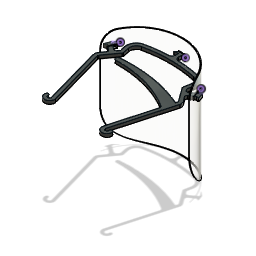
Full_Face_Shield_2.1 (Autodesk Fusion 360 design; units mm, degrees)
Autodesk Fusion 360 part; units mm, degrees
note: some values were not read from the file. Chosen so that the rebuilt part matches the saved one: which face or edge a step refers to; which pieces of a blend or face edit are solid. Set by a fixed rule: which sketch regions a step uses.
(part 1 of 2)
sketch "Sketch1" plane through (0, 0, 0) normal (0, 1, 0) x (1, 0, 0)
  line L0 (0, 0) -> (150, 0) construction
  line L1 (150, 0) -> (150, 165) construction
  line L2 (0, 165) -> (0, 0) construction
  line L3 (75, 0) -> (110, 0) construction
  line L4 (75, 0) -> (40, 0) construction
  line L5 (150, 165) -> (150, 115)
  line L6 (0, 165) -> (0, 115) construction
  line L7 (75, 165) -> (15, 165) construction
  line L8 (16.018879, 159.905605) -> (19.543063, 142.284685)
  line L9 (18.544504, 138.180629) -> (1.725632, 117.15704)
  line L10 (77.5, 165) -> (135, 165)
  line L11 (133.981121, 159.905605) -> (130.456937, 142.284685)
  line L12 (131.455496, 138.180629) -> (148.274368, 117.15704)
  arc A0 (20.165444, 165.82865) -> (16.018879, 159.905605) centre (20.921782, 160.886186) ccw
  arc A1 (133.981121, 159.905605) -> (129.834556, 165.82865) centre (129.078218, 160.886186) ccw
  arc A2 (18.544504, 138.180629) -> (19.543063, 142.284685) centre (14.64016, 141.304105) ccw
  arc A3 (130.456937, 142.284685) -> (131.455496, 138.180629) centre (135.35984, 141.304105) ccw
  arc A4 (1.725632, 117.15704) -> (0.907492, 112.390961) centre (5.629976, 114.033564) ccw
  arc A5 (149.092508, 112.390961) -> (148.274368, 117.15704) centre (144.370024, 114.033564) ccw
  arc A6 (-2.178712, 120.280515) -> (-3.814992, 110.748358) centre (5.629976, 114.033564) ccw
  line L13 (14.64016, 141.304105) -> (-2.178712, 120.280515)
  line L14 (11.115976, 158.925025) -> (14.64016, 141.304105)
  arc A7 (19.409105, 170.771114) -> (11.115976, 158.925025) centre (20.921782, 160.886186) ccw
  arc A8 (130.590895, 170.771114) -> (19.409105, 170.771114) centre (75, -192.5) ccw
  arc A9 (138.884024, 158.925025) -> (130.590895, 170.771114) centre (129.078218, 160.886186) ccw
  line L15 (138.884024, 158.925025) -> (135.35984, 141.304105)
  line L16 (135.35984, 141.304105) -> (152.178712, 120.280515)
  arc A10 (153.814992, 110.748358) -> (152.178712, 120.280515) centre (144.370024, 114.033564) ccw
  line L17 (75, 170) -> (75, 165) construction
  arc A11 (29.826985, 93.888373) -> (50.996347, 169.204402) centre (0.850567, 142.665976) ccw
  arc A12 (42.173763, 96.800594) -> (56.437117, 169.524404) centre (0.850567, 142.665976) ccw
  arc A13 (99.003653, 169.204402) -> (120.173015, 93.888373) centre (149.149433, 142.665976) ccw
  arc A14 (93.562883, 169.524404) -> (107.826237, 96.800594) centre (149.149433, 142.665976) ccw
  circle A15 centre (1.813222, 102.177115) radius 2.5
  circle A16 centre (148.186778, 102.177115) radius 2.5
  line L18 (-3.814992, 110.748358) -> (0, 99.780255)
  line L19 (0.907492, 112.390961) -> (4.174464, 102.998416)
  line L20 (149.092508, 112.390961) -> (145.825536, 102.998416)
  line L21 (153.814992, 110.748358) -> (150, 99.780255)
  arc A17 (145.355882, 79.248283) -> (4.644118, 79.248283) centre (75, -70) ccw
  line L22 (-2.880043, 72.125873) -> (30, -50)
  arc A18 (30, -50) -> (34.828079, -48.700133) centre (32.414039, -49.350066) ccw
  arc A19 (2.512122, 83.770958) -> (-2.880043, 72.125873) centre (6.776115, 74.725608) ccw
  arc A20 (4.644118, 79.248283) -> (1.948036, 73.42574) centre (6.776115, 74.725608) ccw
  line L23 (1.948036, 73.42574) -> (34.828079, -48.700133)
  arc A21 (29.826985, 93.888373) -> (2.512122, 83.770958) centre (75, -70) ccw
  arc A22 (147.487878, 83.770958) -> (120.173015, 93.888373) centre (75, -70) ccw
  arc A23 (50.996347, 169.204402) -> (20.165444, 165.82865) centre (75, -192.5) ccw
  arc A24 (129.834556, 165.82865) -> (99.003653, 169.204402) centre (75, -192.5) ccw
  line L24 (77.5, 170) -> (77.5, 165)
  line L25 (72.5, 165) -> (72.5, 100)
  line L26 (72.5, 100) -> (72.5, 99.500001)
  line L27 (72.5, 99.500001) -> (72.000001, 99.500001)
  line L28 (72.000001, 99.500001) -> (71.807399, 99.500001)
  line L29 (77.5, 165) -> (77.5, 99.500001)
  line L30 (72.5, 165) -> (72.5, 170.500003)
  line L31 (77.5, 169.991379) -> (77.5, 170.500003)
  arc A25 (93.562883, 169.524404) -> (77.5, 169.991379) centre (75, -192.5) ccw
  arc A26 (72.5, 169.991379) -> (56.437117, 169.524404) centre (75, -192.5) ccw
  line L32 (150, 165) -> (77.5, 165) construction
  line L33 (75, 165) -> (0, 165) construction
  arc A27 (107.826237, 96.800594) -> (77.5, 99.981617) centre (75, -70) ccw
  arc A28 (72.5, 99.981617) -> (42.173763, 96.800594) centre (75, -70) ccw
  arc A29 (152.880043, 72.125873) -> (147.487878, 83.770958) centre (143.223885, 74.725608) ccw
  arc A30 (148.051964, 73.42574) -> (145.355882, 79.248283) centre (143.223885, 74.725608) ccw
  line L34 (148.051964, 73.42574) -> (115.171921, -48.700133)
  line L35 (152.880043, 72.125873) -> (120, -50)
  arc A31 (145.355882, 79.248283) -> (4.644118, 79.248283) centre (75, -70) ccw
  arc A32 (115.171921, -48.700133) -> (120, -50) centre (117.585961, -49.350066) ccw
  dimension "d1" = 150
  dimension "d2" = 165
  dimension "d3" = 35
  dimension "d4" = 35
  dimension "d5" = 50
  dimension "d6" = 50
  dimension "d7" = 60
  dimension "d8" = 60
  dimension "d9" = 5
  dimension "d14" = 10
  dimension "d15" = -2.5
  constraint horizontal L0
  constraint vertical L1
  constraint horizontal L32
  constraint vertical L2
  constraint coincident L0.start L2.end
  constraint midpoint L0 L3.start
  constraint parallel L0 L3
  constraint parallel L0 L4
  constraint perpendicular L5 L32
  constraint perpendicular L6 L32
  constraint parallel L7 L32
  constraint parallel L10 L32
  constraint coincident L7.end L8
  constraint coincident L7.end A24
  constraint tangent A0 A24
  constraint tangent L8 A0
  constraint coincident L10.end L11
  constraint coincident L10.end A24
  constraint tangent A1 A24
  constraint tangent L11 A1
  constraint equal A0 A1
  constraint tangent L8 A2
  constraint tangent L9 A2
  constraint equal A0 A2
  constraint tangent L11 A3
  constraint tangent L12 A3
  constraint equal A0 A3
  constraint coincident L6.end L9
  constraint coincident L6.end L19
  constraint tangent L9 A4
  constraint tangent A4 L19
  constraint equal A0 A4
  constraint coincident L5.end L12
  constraint coincident L5.end L20
  constraint tangent L12 A5
  constraint tangent A5 L20
  constraint equal A0 A5
  constraint perpendicular L17 L32
  constraint symmetric L17 A11 A13
  constraint symmetric L17 A12 A14
  constraint tangent A15 L19
  constraint symmetric L17 A15 A16
  constraint parallel L18 L19
  constraint concentric A4 A6
  constraint parallel L9 L13
  constraint parallel L8 L14
  constraint concentric A0 A7
  constraint concentric A8 A24
  constraint concentric A1 A9
  constraint parallel L11 L15
  constraint parallel L12 L16
  constraint concentric A5 A10
  constraint parallel L20 L21
  constraint tangent A6 L18
  constraint tangent L14 A7
  constraint tangent A7 A8
  constraint tangent A6 L13
  constraint tangent A9 L15
  constraint tangent A8 A9
  constraint tangent L16 A10
  constraint tangent A10 L21
  constraint concentric A17 A22
  constraint tangent A19 A22
  constraint tangent L22 A19
  constraint concentric A11 A12
  constraint concentric A21 A22
  constraint concentric A19 A20
  constraint parallel L22 L23
  constraint tangent A20 L23
  constraint concentric A22 A27
  constraint concentric A23 A24
  constraint coincident L17.start A24
  constraint concentric A24 A25
  constraint parallel L25 L26
  constraint perpendicular L26 L27
  constraint perpendicular L26 L28
  constraint perpendicular L27 L29
  constraint parallel L25 L30
  constraint parallel L25 L31
  constraint concentric A25 A26
  constraint collinear L32 L33
  constraint coincident L7.start L32
  constraint concentric A27 A28
  constraint symmetric L17 L22.end L35.end
  constraint symmetric L17 A19 A29
  constraint symmetric L17 A20 A30
  constraint tangent L35 A32
  measures "d1" distance of L0.start L0.end
  measures "d2" distance of L0.start L2.start
  measures "d3" distance of L3.start L3.end
  measures "d4" distance of L3.start L4.end
  measures "d5" distance of L1.end L5.end
  measures "d6" distance of L2.start L6.end
  measures "d7" distance of L7.start L7.end
  measures "d8" distance of L7.start L10.end
  measures "d9" radius of A0
  measures "d14" radius of A19
sketch "Sketch2" plane through (0, 0, 0) normal (0, 1, 0) x (1, 0, 0)
  arc A0 (74.500001, 175.000338) -> (20, 171.000003) centre (74.500001, -198.250003) ccw
  arc A1 (74.500001, 170.000338) -> (20.730073, 166.05359) centre (74.500001, -198.250003) ccw
  arc A2 (20, 171.000003) -> (11, 159.000002) centre (20.833334, 161.000002) ccw
  line L0 (11, 159.000002) -> (14.161452, 143.4562)
  line L1 (13.13349, 139.295831) -> (-1, 122.000002)
  arc A3 (-1, 122.000002) -> (-3.968884, 110.553272) centre (7.879032, 113.588711) ccw
  line L2 (0.330661, 92.053201) -> (30, -50)
  arc A4 (0.330661, 92.053201) -> (-3.968884, 110.553272) centre (-413.734399, 5.571259) ccw
  arc A5 (30, -50) -> (34.894386, -48.977755) centre (32.447193, -49.488877) ccw
  arc A6 (114.105616, -48.977755) -> (119.000002, -50) centre (116.552809, -49.488877) ccw
  arc A7 (13.13349, 139.295831) -> (14.161452, 143.4562) centre (9.261768, 142.459654) ccw
  arc A8 (20.415228, 166.017274) -> (15.899683, 159.996548) centre (20.833334, 161.000002) ccw
  line L3 (15.899683, 159.996548) -> (19.061135, 144.452745)
  arc A9 (17.005211, 136.132009) -> (19.061135, 144.452745) centre (9.261768, 142.459654) ccw
  line L4 (17.005211, 136.132009) -> (2.74065, 118.675781)
  arc A10 (2.74065, 118.675781) -> (0.87468, 111.794195) centre (7.879032, 113.588711) ccw
  arc A11 (5.225047, 93.075446) -> (0.87468, 111.794195) centre (-413.734399, 5.571259) ccw
  line L5 (5.225047, 93.075446) -> (34.894386, -48.977755)
  line L6 (20.415228, 166.017274) -> (20.730073, 166.05359)
  arc A12 (138.000002, 159.000002) -> (129.000002, 171.000003) centre (128.166669, 161.000002) ccw
  line L7 (133.100319, 159.996548) -> (129.938867, 144.452745)
  line L8 (128.584775, 166.017274) -> (128.269929, 166.05359)
  arc A13 (134.838551, 143.4562) -> (135.866513, 139.295831) centre (139.738234, 142.459654) ccw
  arc A14 (129.938867, 144.452745) -> (131.994791, 136.132009) centre (139.738234, 142.459654) ccw
  line L9 (135.866513, 139.295831) -> (150.000002, 122.000002)
  line L10 (138.000002, 159.000002) -> (134.838551, 143.4562)
  arc A15 (129.000002, 171.000003) -> (74.500001, 175.000338) centre (74.500001, -198.250003) ccw
  arc A16 (128.269929, 166.05359) -> (74.500001, 170.000338) centre (74.500001, -198.250003) ccw
  line L11 (131.994791, 136.132009) -> (146.259352, 118.675781)
  arc A17 (133.100319, 159.996548) -> (128.584775, 166.017274) centre (128.166669, 161.000002) ccw
  arc A18 (114.105616, -48.977755) -> (119.000002, -50) centre (116.552809, -49.488877) ccw
  arc A19 (148.125323, 111.794195) -> (146.259352, 118.675781) centre (141.12097, 113.588711) ccw
  arc A20 (152.968887, 110.553272) -> (148.669341, 92.053201) centre (562.734401, 5.571259) ccw
  line L12 (148.669341, 92.053201) -> (119.000002, -50)
  arc A21 (152.968887, 110.553272) -> (150.000002, 122.000002) centre (141.12097, 113.588711) ccw
  arc A22 (141.330243, 87.437278) -> (20, 105) centre (60.923824, -40.162066) ccw
  arc A23 (18.643293, 109.812416) -> (20, 105) centre (19.321646, 107.406208) ccw
  arc A24 (144.508875, 105.691884) -> (38.867306, 114.089347) centre (73.772595, -115.489468) ccw
  arc A25 (143.77951, 100.674062) -> (103.197421, 109.81437) centre (73.772595, -115.489468) ccw
  arc A26 (141.247218, 93.359995) -> (103.197421, 109.81437) centre (60.923824, -40.162066) ccw
  arc A27 (38.867306, 114.089347) -> (18.643293, 109.812416) centre (60.923824, -40.162066) ccw
  arc A28 (148.125323, 111.794195) -> (146.939836, 107.054655) centre (562.734401, 5.571259) ccw
  line L13 (142.179397, 85.436106) -> (114.105616, -48.977755)
  arc A29 (144.941934, 98.487642) -> (143.678642, 100.710483) centre (143.082367, 98.901207) ccw
  arc A30 (141.247218, 93.359995) -> (144.093982, 94.602909) centre (142.229221, 94.992385) ccw
  arc A31 (142.179397, 85.436106) -> (141.330243, 87.437278) centre (140.314636, 85.825581) ccw
  arc A32 (144.508875, 105.691884) -> (146.939836, 107.054655) centre (145.089162, 107.506351) ccw
  line L14 (144.941934, 98.487642) -> (144.093982, 94.602909)
  point P0 (149.000002, 0)
  dimension "d17" = -5
  dimension "d18" = 423
  dimension "d19" = -5
  dimension "d20" = 5
  dimension "d23" = 1.905
  dimension "d24" = 1.905
  dimension "d25" = 1.905
  constraint tangent A2 L0
  constraint tangent A3 A4
  constraint tangent L2 A4
  constraint tangent A5 L5
  constraint tangent A22 A23
  constraint concentric A22 A26
  constraint concentric A24 A25
  constraint concentric A26 A27
  constraint tangent A26 A30
  constraint equal A29 A30
  constraint tangent A22 A31
  constraint tangent L13 A31
  constraint tangent A24 A32
  constraint tangent A28 A32
  measures "d18" radius of A4
  measures "d20" radius of A7
  measures "d23" radius of A29
  measures "d24" radius of A31
  measures "d25" radius of A32
sketch "Sketch3" plane through (0, 0, 0) normal (0, 1, 0) x (1, 0, 0)
  arc A0 (143.161124, 90.146177) -> (22.481496, 123.208852) centre (28.068159, -93.172915) ccw
  arc A1 (151.469892, 109.695095) -> (21.748345, 130.644222) centre (45.713045, -133.067717) ccw
  line L0 (15.075976, 155.760128) -> (17.56166, 143.33171)
  line L1 (17.125174, 141.339618) -> (-1.860243, 115.234669)
  line L2 (-2.25178, 113.05513) -> (50.799999, -76.199999)
  line L3 (75.106127, 175.000109) -> (75.106127, 157.480005) construction
  line L4 (135.136278, 155.760128) -> (132.650594, 143.33171)
  line L5 (133.08708, 141.339618) -> (152.034083, 115.287488)
  arc A2 (125.422656, 170.65176) -> (24.789597, 170.65176) centre (75.106127, -57.096199) ccw
  arc A3 (24.789597, 170.65176) -> (15.075976, 155.760128) centre (27.52935, 158.250803) ccw
  arc A4 (135.136278, 155.760128) -> (125.422656, 170.65176) centre (122.682903, 158.250803) ccw
  arc A5 (17.125174, 141.339618) -> (17.56166, 143.33171) centre (15.070985, 142.833575) ccw
  arc A6 (132.650594, 143.33171) -> (133.08708, 141.339618) centre (135.141269, 142.833575) ccw
  arc A7 (-1.860243, 115.234669) -> (-2.25178, 113.05513) centre (0.193946, 113.740713) ccw
  arc A8 (152.425798, 113.108587) -> (152.034083, 115.287488) centre (149.979894, 113.793532) ccw
  line L6 (-8.366095, 111.341172) -> (44.685684, -77.913957)
  arc A9 (-6.995717, 118.96956) -> (-8.366095, 111.341172) centre (0.193946, 113.740713) ccw
  line L7 (8.849289, 154.51479) -> (11.007461, 143.72393)
  arc A10 (23.419721, 176.852239) -> (8.849289, 154.51479) centre (27.52935, 158.250803) ccw
  arc A11 (126.792533, 176.852239) -> (23.419721, 176.852239) centre (75.106127, -57.096199) ccw
  arc A12 (141.362965, 154.51479) -> (126.792533, 176.852239) centre (122.682903, 158.250803) ccw
  line L8 (141.362965, 154.51479) -> (139.204793, 143.72393)
  arc A13 (158.54056, 111.396223) -> (157.169557, 119.022379) centre (149.979894, 113.793532) ccw
  line L9 (158.54056, 111.396223) -> (105.527016, -77.912363)
  arc A14 (99.412255, -76.199999) -> (105.527016, -77.912363) centre (102.469636, -77.056181) ccw
  arc A15 (44.685684, -77.913957) -> (50.799999, -76.199999) centre (47.742842, -77.056978) ccw
  line L10 (152.425798, 113.108587) -> (151.469892, 109.695095)
  line L11 (144.804126, 85.891994) -> (99.412255, -76.199999)
  arc A16 (10.384163, 0.007596) -> (29.434159, 0.019779) centre (19.910098, -1.451354) ccw
  arc A17 (16.660973, -0.953733) -> (23.158584, -0.949577) centre (19.910098, -1.451354) ccw
  arc A18 (16.660973, -0.953733) -> (10.384163, 0.007596) centre (13.522568, -0.473068) ccw
  arc A19 (120.778095, 0.019779) -> (139.828091, 0.007596) centre (130.302156, -1.451354) ccw
  arc A20 (127.053671, -0.949575) -> (133.55128, -0.953733) centre (130.302156, -1.451354) ccw
  arc A21 (139.828091, 0.007596) -> (133.55128, -0.953733) centre (136.689686, -0.473068) ccw
  line L12 (120.778095, 0.019779) -> (120.850229, 0.353884)
  line L13 (-12.339129, 150.464332) -> (-16.304061, 138.860017)
  line L14 (-1.075524, 133.587526) -> (-11.019318, 140.819377)
  line L15 (-12.671259, 137.201336) -> (-11.019318, 140.819377)
  line L16 (3.039912, 139.24625) -> (-9.700548, 148.512039)
  line L17 (-16.304061, 138.860017) -> (-12.671259, 137.201336)
  line L18 (11.007461, 143.72393) -> (8.36213, 140.0866)
  line L19 (-0.235173, 128.265308) -> (-6.995717, 118.96956)
  arc A22 (-0.235173, 128.265308) -> (-1.075524, 133.587526) centre (-3.316458, 130.506242) ccw
  arc A23 (3.039912, 139.24625) -> (8.36213, 140.0866) centre (5.280846, 142.327534) ccw
  arc A24 (23.319068, 130.782246) -> (23.41734, 123.230989) centre (22.860001, 127.000004) ccw
  arc A25 (141.850124, 140.0866) -> (147.172342, 139.24625) centre (144.931408, 142.327534) ccw
  arc A26 (151.287777, 133.587526) -> (150.447427, 128.265308) centre (153.528712, 130.506242) ccw
  line L20 (151.287777, 133.587526) -> (161.231572, 140.819377)
  line L21 (147.172342, 139.24625) -> (159.912802, 148.512039)
  line L22 (166.516315, 138.860017) -> (162.883513, 137.201336)
  line L23 (162.551383, 150.464332) -> (166.516315, 138.860017)
  line L24 (162.883513, 137.201336) -> (161.231572, 140.819377)
  line L25 (139.204793, 143.72393) -> (141.850124, 140.0866)
  line L26 (150.447427, 128.265308) -> (157.169557, 119.022379)
  arc A27 (144.804126, 85.891994) -> (143.161124, 90.146177) centre (141.135269, 86.919412) ccw
  line L27 (-9.700548, 148.512039) -> (-2.54, 157.480005)
  line L28 (-2.54, 157.480005) -> (-3.330318, 158.111041)
  line L29 (-3.330318, 158.111041) -> (-12.339129, 150.464332)
  line L30 (159.912802, 148.512039) -> (152.752254, 157.480005)
  line L31 (153.542572, 158.111041) -> (162.551383, 150.464332)
  line L32 (152.752254, 157.480005) -> (153.542572, 158.111041)
  dimension "d26" = 7.62
  dimension "d27" = 12.7
  dimension "d28" = 2.54
  dimension "d32" = 19.05
  dimension "d33" = -6.35
  dimension "d41" = 3.81
  dimension "d42" = 3.81
  constraint vertical L3
  constraint tangent A2 A3
  constraint tangent L0 A3
  constraint tangent A2 A4
  constraint tangent L4 A4
  constraint equal A3 A4
  constraint tangent L0 A5
  constraint tangent L1 A5
  constraint tangent L4 A6
  constraint tangent L5 A6
  constraint equal A5 A6
  constraint tangent L1 A7
  constraint tangent L2 A7
  constraint equal A5 A7
  constraint tangent L5 A8
  constraint tangent A8 L10
  constraint equal A5 A8
  constraint tangent L2 A15
  constraint collinear L10 L11
  constraint parallel L2 L6
  constraint concentric A7 A9
  constraint parallel L1 L18
  constraint parallel L0 L7
  constraint concentric A3 A10
  constraint concentric A2 A11
  constraint concentric A4 A12
  constraint parallel L4 L8
  constraint parallel L5 L25
  constraint concentric A8 A13
  constraint tangent L7 A10
  constraint tangent A10 A11
  constraint tangent A13 L9
  constraint tangent A11 A12
  constraint tangent A12 L8
  constraint tangent A13 L25
  constraint tangent A17 A18
  constraint symmetric L3 A16 A19
  constraint symmetric L3 A17 A20
  constraint symmetric L3 A18 A21
  constraint perpendicular L14 L18
  constraint perpendicular L16 L18
  constraint perpendicular L15 L17
  constraint collinear L18 L19
  constraint tangent L19 A22
  constraint tangent L14 A22
  constraint tangent L16 A23
  constraint tangent L18 A23
  constraint equal A22 A23
  constraint symmetric L3 A22 A26
  constraint symmetric L3 A23 A25
  constraint collinear L25 L26
  constraint tangent A0 A27
  constraint tangent L11 A27
  constraint perpendicular L27 L28
  measures "d26" diameter of A24
  measures "d27" radius of A3
  measures "d28" radius of A5
  measures "d41" radius of A22
  measures "d42" radius of A27
extrude "Extrude1" add sketch "Sketch3" along normal blind 6.223 contours A0 A1 L0 L1 L2 L4 L5 A2 A3 A4 A5 A6 A7 A8 L6 A9 L7 A10 A11 A12 L8 A13 L9 L10 L11 A16 A19 L12 L13 L14 L15 L16 L17 L18 L19 A22 A23 A24 A25 A26 L20 L21 L22 L23 L24 L25 L26 A27 L27 L28 L29 L30 L31 L32 | A1 A24 picked at (136.663738, 101.580003) picked at (22.616663, 130.769907) makes body 1
sketch "Sketch4" plane through (0, 6.223, 0) normal (0, 1, 0) x (-1, 0, 0)
  arc A0 (-143.161124, -90.146177) -> (-22.481496, -123.208852) centre (-28.068159, 93.172915) ccw
  line L0 (-144.804126, -85.891994) -> (-120.850229, -0.353884)
  line L1 (-124.735935, 9.318321) -> (-158.54056, -111.396223)
  arc A1 (-158.54056, -111.396223) -> (-157.169557, -119.022379) centre (-149.979894, -113.793532) ccw
  line L2 (-157.169557, -119.022379) -> (-150.447427, -128.265308)
  line L3 (-139.204793, -143.72393) -> (-141.362965, -154.51479)
  arc A2 (-141.362965, -154.51479) -> (-126.792533, -176.852239) centre (-122.682903, -158.250803) ccw
  arc A3 (-126.792533, -176.852239) -> (-23.419721, -176.852239) centre (-75.106127, 57.096199) ccw
  arc A4 (-23.419721, -176.852239) -> (-8.849289, -154.51479) centre (-27.52935, -158.250803) ccw
  line L4 (-8.849289, -154.51479) -> (-11.007461, -143.72393)
  line L5 (-11.007461, -143.72393) -> (-8.36213, -140.0866)
  arc A5 (6.995717, -118.96956) -> (8.366095, -111.341172) centre (-0.193946, -113.740713) ccw
  line L6 (8.366095, -111.341172) -> (-25.460221, 9.329686)
  line L7 (-29.434159, -0.019779) -> (2.25178, -113.05513)
  arc A6 (1.860243, -115.234669) -> (2.25178, -113.05513) centre (-0.193946, -113.740713) ccw
  line L8 (1.860243, -115.234669) -> (-17.125174, -141.339618)
  arc A7 (-17.125174, -141.339618) -> (-17.56166, -143.33171) centre (-15.070985, -142.833575) ccw
  line L9 (-17.56166, -143.33171) -> (-15.075976, -155.760128)
  arc A8 (-24.789597, -170.65176) -> (-15.075976, -155.760128) centre (-27.52935, -158.250803) ccw
  arc A9 (-125.422656, -170.65176) -> (-24.789597, -170.65176) centre (-75.106127, 57.096199) ccw
  arc A10 (-135.136278, -155.760128) -> (-125.422656, -170.65176) centre (-122.682903, -158.250803) ccw
  line L10 (-135.136278, -155.760128) -> (-132.650594, -143.33171)
  arc A11 (-132.650594, -143.33171) -> (-133.08708, -141.339618) centre (-135.141269, -142.833575) ccw
  line L11 (-133.08708, -141.339618) -> (-152.034083, -115.287488)
  arc A12 (-152.425798, -113.108587) -> (-152.034083, -115.287488) centre (-149.979894, -113.793532) ccw
  line L12 (-152.425798, -113.108587) -> (-151.469892, -109.695095)
  arc A13 (-151.469892, -109.695095) -> (-23.319068, -130.782246) centre (-45.713045, 133.067717) ccw
  arc A14 (-23.319068, -130.782246) -> (-22.481496, -123.208852) centre (-22.860001, -127.000004) ccw
  arc A15 (-144.804126, -85.891994) -> (-143.161124, -90.146177) centre (-141.135269, -86.919412) ccw
  line L13 (-120.850229, -0.353884) -> (-120.778095, -0.019779)
  arc A16 (-120.778095, -0.019779) -> (-124.735935, 9.318321) centre (-130.302156, 1.451354) ccw
  arc A17 (-151.287777, -133.587526) -> (-150.447427, -128.265308) centre (-153.528712, -130.506242) ccw
  line L14 (-151.287777, -133.587526) -> (-161.231572, -140.819377)
  line L15 (-161.231572, -140.819377) -> (-162.883513, -137.201336)
  line L16 (-162.883513, -137.201336) -> (-166.516315, -138.860017)
  line L17 (-166.516315, -138.860017) -> (-162.551383, -150.464332)
  line L18 (-159.912802, -148.512039) -> (-147.172342, -139.24625)
  arc A18 (-141.850124, -140.0866) -> (-147.172342, -139.24625) centre (-144.931408, -142.327534) ccw
  line L19 (-141.850124, -140.0866) -> (-139.204793, -143.72393)
  arc A19 (-3.039912, -139.24625) -> (-8.36213, -140.0866) centre (-5.280846, -142.327534) ccw
  line L20 (-3.039912, -139.24625) -> (9.700548, -148.512039)
  line L21 (12.339129, -150.464332) -> (16.304061, -138.860017)
  line L22 (16.304061, -138.860017) -> (12.671259, -137.201336)
  line L23 (12.671259, -137.201336) -> (11.019318, -140.819377)
  line L24 (11.019318, -140.819377) -> (1.075524, -133.587526)
  arc A20 (0.235173, -128.265308) -> (1.075524, -133.587526) centre (3.316458, -130.506242) ccw
  line L25 (0.235173, -128.265308) -> (6.995717, -118.96956)
  arc A21 (-25.460221, 9.329686) -> (-29.434159, -0.019779) centre (-19.910098, 1.451354) ccw
  line L26 (-162.551383, -150.464332) -> (-153.542572, -158.111041)
  line L27 (-153.542572, -158.111041) -> (-152.752254, -157.480005)
  line L28 (-152.752254, -157.480005) -> (-159.912802, -148.512039)
  line L29 (9.700548, -148.512039) -> (2.54, -157.480005)
  line L30 (2.54, -157.480005) -> (3.330318, -158.111041)
  line L31 (3.330318, -158.111041) -> (12.339129, -150.464332)
sketch "Sketch6" plane through (0, 6.223, 0) normal (0, 1, 0) x (-1, 0, 0)
sketch "Sketch7" plane through (0, 0, 0) normal (0, 1, 0) x (1, 0, 0)
extrude "Extrude2" add sketch "Sketch3" along normal blind 6.096 separate body contours A0 A1 L0 L1 L2 L4 L5 A2 A3 A4 A5 A6 A7 A8 L6 A9 L7 A10 A11 A12 L8 A13 L9 L10 L11 A16 A19 L12 L13 L14 L15 L16 L17 L18 L19 A22 A23 A24 A25 A26 L20 L21 L22 L23 L24 L25 L26 A27 L27 L28 L29 L30 L31 L32 | L9 A19 A20 A21 | L6 A16 A17 A18 picked at (136.663738, 101.580003) picked at (136.737423, 1.155029) picked at (12.864675, 0.355935) makes body 2
sketch "Sketch8" plane through (0, 0, 0) normal (0, -1, 0) x (1, 0, 0)
  arc A0 (139.828091, -0.007596) -> (120.778095, -0.019779) centre (130.302156, 1.451354) ccw
  line L0 (120.778095, -0.019779) -> (120.850229, -0.353884)
  line L1 (120.850229, -0.353884) -> (144.804126, -85.891994)
  arc A1 (22.481496, -123.208852) -> (143.161124, -90.146177) centre (28.068159, 93.172915) ccw
  arc A2 (22.481496, -123.208852) -> (21.748345, -130.644222) centre (22.860001, -127.000004) ccw
  arc A3 (21.748345, -130.644222) -> (151.469892, -109.695095) centre (45.713045, 133.067717) ccw
  line L2 (151.469892, -109.695095) -> (152.425798, -113.108587)
  arc A4 (152.034083, -115.287488) -> (152.425798, -113.108587) centre (149.979894, -113.793532) ccw
  line L3 (152.034083, -115.287488) -> (133.08708, -141.339618)
  arc A5 (133.08708, -141.339618) -> (132.650594, -143.33171) centre (135.141269, -142.833575) ccw
  line L4 (132.650594, -143.33171) -> (135.136278, -155.760128)
  arc A6 (125.422656, -170.65176) -> (135.136278, -155.760128) centre (122.682903, -158.250803) ccw
  arc A7 (24.789597, -170.65176) -> (125.422656, -170.65176) centre (75.106127, 57.096199) ccw
  arc A8 (15.075976, -155.760128) -> (24.789597, -170.65176) centre (27.52935, -158.250803) ccw
  line L5 (15.075976, -155.760128) -> (17.56166, -143.33171)
  arc A9 (17.56166, -143.33171) -> (17.125174, -141.339618) centre (15.070985, -142.833575) ccw
  line L6 (17.125174, -141.339618) -> (-1.860243, -115.234669)
  arc A10 (-2.25178, -113.05513) -> (-1.860243, -115.234669) centre (0.193946, -113.740713) ccw
  line L7 (-2.25178, -113.05513) -> (29.434159, -0.019779)
  arc A11 (29.434159, -0.019779) -> (10.384163, -0.007596) centre (19.910098, 1.451354) ccw
  arc A12 (10.384163, -0.007596) -> (16.660973, 0.953733) centre (13.522568, 0.473068) ccw
  arc A13 (23.189622, 1.229628) -> (16.660973, 0.953733) centre (19.910098, 1.451354) ccw
  line L8 (23.189622, 1.229628) -> (-8.366095, -111.341172)
  arc A14 (-8.366095, -111.341172) -> (-6.995717, -118.96956) centre (0.193946, -113.740713) ccw
  line L9 (-6.995717, -118.96956) -> (-0.235173, -128.265308)
  line L10 (11.007461, -143.72393) -> (8.849289, -154.51479)
  arc A15 (8.849289, -154.51479) -> (23.419721, -176.852239) centre (27.52935, -158.250803) ccw
  arc A16 (23.419721, -176.852239) -> (126.792533, -176.852239) centre (75.106127, 57.096199) ccw
  arc A17 (126.792533, -176.852239) -> (141.362965, -154.51479) centre (122.682903, -158.250803) ccw
  line L11 (141.362965, -154.51479) -> (139.204793, -143.72393)
  line L12 (139.204793, -143.72393) -> (141.850124, -140.0866)
  arc A18 (157.169557, -119.022379) -> (158.54056, -111.396223) centre (149.979894, -113.793532) ccw
  line L13 (158.54056, -111.396223) -> (127.031955, 1.119355)
  arc A19 (133.55128, 0.953733) -> (127.031955, 1.119355) centre (130.302156, 1.451354) ccw
  arc A20 (133.55128, 0.953733) -> (139.828091, -0.007596) centre (136.689686, 0.473068) ccw
  arc A21 (143.161124, -90.146177) -> (144.804126, -85.891994) centre (141.135269, -86.919412) ccw
  arc A22 (-1.075524, -133.587526) -> (-0.235173, -128.265308) centre (-3.316458, -130.506242) ccw
  line L14 (-1.075524, -133.587526) -> (-11.019318, -140.819377)
  line L15 (-11.019318, -140.819377) -> (-12.671259, -137.201336)
  line L16 (-12.671259, -137.201336) -> (-16.304061, -138.860017)
  line L17 (-16.304061, -138.860017) -> (-12.339129, -150.464332)
  line L18 (-9.700548, -148.512039) -> (3.039912, -139.24625)
  arc A23 (8.36213, -140.0866) -> (3.039912, -139.24625) centre (5.280846, -142.327534) ccw
  line L19 (8.36213, -140.0866) -> (11.007461, -143.72393)
  arc A24 (147.172342, -139.24625) -> (141.850124, -140.0866) centre (144.931408, -142.327534) ccw
  line L20 (147.172342, -139.24625) -> (159.912802, -148.512039)
  line L21 (162.551383, -150.464332) -> (166.516315, -138.860017)
  line L22 (166.516315, -138.860017) -> (162.883513, -137.201336)
  line L23 (162.883513, -137.201336) -> (161.231572, -140.819377)
  line L24 (161.231572, -140.819377) -> (151.287777, -133.587526)
  arc A25 (150.447427, -128.265308) -> (151.287777, -133.587526) centre (153.528712, -130.506242) ccw
  line L25 (150.447427, -128.265308) -> (157.169557, -119.022379)
  line L26 (-12.339129, -150.464332) -> (-3.330318, -158.111041)
  line L27 (-3.330318, -158.111041) -> (-2.54, -157.480005)
  line L28 (-2.54, -157.480005) -> (-9.700548, -148.512039)
  line L29 (159.912802, -148.512039) -> (152.752254, -157.480005)
  line L30 (152.752254, -157.480005) -> (153.542572, -158.111041)
  line L31 (153.542572, -158.111041) -> (162.551383, -150.464332)
sketch "Sketch9" plane through (0, 0, 0) normal (0, -1, 0) x (1, 0, 0)
sketch "Sketch10" plane through (0, 0, 0) normal (0, -1, 0) x (1, 0, 0)
  arc A0 (139.828091, -0.007596) -> (120.778095, -0.019779) centre (130.302156, 1.451354) ccw
  line L0 (120.778095, -0.019779) -> (120.850229, -0.353884)
  line L1 (120.850229, -0.353884) -> (144.804126, -85.891994)
  arc A1 (143.161124, -90.146177) -> (144.804126, -85.891994) centre (141.135269, -86.919412) ccw
  arc A2 (22.481496, -123.208852) -> (143.161124, -90.146177) centre (28.068159, 93.172915) ccw
  arc A3 (22.481496, -123.208852) -> (21.748345, -130.644222) centre (22.860001, -127.000004) ccw
  arc A4 (21.748345, -130.644222) -> (151.469892, -109.695095) centre (45.713045, 133.067717) ccw
  line L2 (151.469892, -109.695095) -> (152.425798, -113.108587)
  arc A5 (152.034083, -115.287488) -> (152.425798, -113.108587) centre (149.979894, -113.793532) ccw
  line L3 (152.034083, -115.287488) -> (133.08708, -141.339618)
  arc A6 (133.08708, -141.339618) -> (132.650594, -143.33171) centre (135.141269, -142.833575) ccw
  line L4 (132.650594, -143.33171) -> (135.136278, -155.760128)
  arc A7 (125.422656, -170.65176) -> (135.136278, -155.760128) centre (122.682903, -158.250803) ccw
  arc A8 (24.789597, -170.65176) -> (125.422656, -170.65176) centre (75.106127, 57.096199) ccw
  arc A9 (15.075976, -155.760128) -> (24.789597, -170.65176) centre (27.52935, -158.250803) ccw
  line L5 (15.075976, -155.760128) -> (17.56166, -143.33171)
  arc A10 (17.56166, -143.33171) -> (17.125174, -141.339618) centre (15.070985, -142.833575) ccw
  line L6 (17.125174, -141.339618) -> (-1.860243, -115.234669)
  arc A11 (-2.25178, -113.05513) -> (-1.860243, -115.234669) centre (0.193946, -113.740713) ccw
  line L7 (-2.25178, -113.05513) -> (29.434159, -0.019779)
  arc A12 (29.434159, -0.019779) -> (10.384163, -0.007596) centre (19.910098, 1.451354) ccw
  arc A13 (10.384163, -0.007596) -> (16.660973, 0.953733) centre (13.522568, 0.473068) ccw
  arc A14 (23.189622, 1.229628) -> (16.660973, 0.953733) centre (19.910098, 1.451354) ccw
  line L8 (23.189622, 1.229628) -> (-8.366095, -111.341172)
  arc A15 (-8.366095, -111.341172) -> (-6.995717, -118.96956) centre (0.193946, -113.740713) ccw
  line L9 (-6.995717, -118.96956) -> (-0.235173, -128.265308)
  arc A16 (-1.075524, -133.587526) -> (-0.235173, -128.265308) centre (-3.316458, -130.506242) ccw
  line L10 (-1.075524, -133.587526) -> (-11.019318, -140.819377)
  line L11 (-11.019318, -140.819377) -> (-12.671259, -137.201336)
  line L12 (-12.671259, -137.201336) -> (-16.304061, -138.860017)
  line L13 (-16.304061, -138.860017) -> (-12.339129, -150.464332)
  line L14 (-9.700548, -148.512039) -> (3.039912, -139.24625)
  arc A17 (8.36213, -140.0866) -> (3.039912, -139.24625) centre (5.280846, -142.327534) ccw
  line L15 (8.36213, -140.0866) -> (11.007461, -143.72393)
  line L16 (11.007461, -143.72393) -> (8.849289, -154.51479)
  arc A18 (8.849289, -154.51479) -> (23.419721, -176.852239) centre (27.52935, -158.250803) ccw
  arc A19 (23.419721, -176.852239) -> (126.792533, -176.852239) centre (75.106127, 57.096199) ccw
  arc A20 (126.792533, -176.852239) -> (141.362965, -154.51479) centre (122.682903, -158.250803) ccw
  line L17 (141.362965, -154.51479) -> (139.204793, -143.72393)
  line L18 (139.204793, -143.72393) -> (141.850124, -140.0866)
  arc A21 (147.172342, -139.24625) -> (141.850124, -140.0866) centre (144.931408, -142.327534) ccw
  line L19 (147.172342, -139.24625) -> (159.912802, -148.512039)
  line L20 (162.551383, -150.464332) -> (166.516315, -138.860017)
  line L21 (166.516315, -138.860017) -> (162.883513, -137.201336)
  line L22 (162.883513, -137.201336) -> (161.231572, -140.819377)
  line L23 (161.231572, -140.819377) -> (151.287777, -133.587526)
  arc A22 (150.447427, -128.265308) -> (151.287777, -133.587526) centre (153.528712, -130.506242) ccw
  line L24 (150.447427, -128.265308) -> (157.169557, -119.022379)
  arc A23 (157.169557, -119.022379) -> (158.54056, -111.396223) centre (149.979894, -113.793532) ccw
  line L25 (158.54056, -111.396223) -> (127.031955, 1.119355)
  arc A24 (133.55128, 0.953733) -> (127.031955, 1.119355) centre (130.302156, 1.451354) ccw
  arc A25 (133.55128, 0.953733) -> (139.828091, -0.007596) centre (136.689686, 0.473068) ccw
  line L26 (-12.339129, -150.464332) -> (-3.330318, -158.111041)
  line L27 (-3.330318, -158.111041) -> (-2.54, -157.480005)
  line L28 (-2.54, -157.480005) -> (-9.700548, -148.512039)
  line L29 (159.912802, -148.512039) -> (152.752254, -157.480005)
  line L30 (152.752254, -157.480005) -> (153.542572, -158.111041)
  line L31 (153.542572, -158.111041) -> (162.551383, -150.464332)
chamfer "Chamfer1" distance 3.81 angle 45 1 edges at (-12.671259, 3.048, -137.201336) on bodies 2
chamfer "Chamfer2" distance 3.81 angle 45 1 edges at (162.883513, 3.048, -137.201336) on bodies 2
sketch "Sketch11" plane through (0, 0, 0) normal (0, 0, 1) x (1, 0, 0)
sketch "Sketch12" plane through (0, 6.096, 0) normal (0, 1, 0) x (-1, 0, 0)
  line L0 (-161.30107, -140.667166) -> (-166.349343, -138.78378)
  line L1 (-166.349343, -138.78378) -> (-166.516315, -138.860017)
  line L2 (-166.516315, -138.860017) -> (-162.551383, -150.464332)
  line L3 (-159.912802, -148.512039) -> (-147.172342, -139.24625)
  arc A0 (-141.850124, -140.0866) -> (-147.172342, -139.24625) centre (-144.931408, -142.327534) ccw
  line L4 (-141.850124, -140.0866) -> (-139.204793, -143.72393)
  line L5 (-139.204793, -143.72393) -> (-141.362965, -154.51479)
  arc A1 (-141.362965, -154.51479) -> (-126.792533, -176.852239) centre (-122.682903, -158.250803) ccw
  arc A2 (-126.792533, -176.852239) -> (-23.419721, -176.852239) centre (-75.106127, 57.096199) ccw
  arc A3 (-23.419721, -176.852239) -> (-8.849289, -154.51479) centre (-27.52935, -158.250803) ccw
  line L6 (-8.849289, -154.51479) -> (-11.007461, -143.72393)
  line L7 (-11.007461, -143.72393) -> (-8.36213, -140.0866)
  arc A4 (-3.039912, -139.24625) -> (-8.36213, -140.0866) centre (-5.280846, -142.327534) ccw
  line L8 (-3.039912, -139.24625) -> (9.700548, -148.512039)
  line L9 (12.339129, -150.464332) -> (16.304061, -138.860017)
  line L10 (16.304061, -138.860017) -> (16.137089, -138.78378)
  line L11 (16.137089, -138.78378) -> (11.088816, -140.667166)
  line L12 (11.088816, -140.667166) -> (11.019318, -140.819377)
  line L13 (11.019318, -140.819377) -> (1.075524, -133.587526)
  arc A5 (0.235173, -128.265308) -> (1.075524, -133.587526) centre (3.316458, -130.506242) ccw
  line L14 (0.235173, -128.265308) -> (6.995717, -118.96956)
  arc A6 (6.995717, -118.96956) -> (8.366095, -111.341172) centre (-0.193946, -113.740713) ccw
  line L15 (8.366095, -111.341172) -> (-23.189622, 1.229628)
  arc A7 (-16.660973, 0.953733) -> (-23.189622, 1.229628) centre (-19.910098, 1.451354) ccw
  arc A8 (-16.660973, 0.953733) -> (-10.384163, -0.007596) centre (-13.522568, 0.473068) ccw
  arc A9 (-10.384163, -0.007596) -> (-29.434159, -0.019779) centre (-19.910098, 1.451354) ccw
  line L16 (-29.434159, -0.019779) -> (2.25178, -113.05513)
  arc A10 (1.860243, -115.234669) -> (2.25178, -113.05513) centre (-0.193946, -113.740713) ccw
  line L17 (1.860243, -115.234669) -> (-17.125174, -141.339618)
  arc A11 (-17.125174, -141.339618) -> (-17.56166, -143.33171) centre (-15.070985, -142.833575) ccw
  line L18 (-17.56166, -143.33171) -> (-15.075976, -155.760128)
  arc A12 (-24.789597, -170.65176) -> (-15.075976, -155.760128) centre (-27.52935, -158.250803) ccw
  arc A13 (-125.422656, -170.65176) -> (-24.789597, -170.65176) centre (-75.106127, 57.096199) ccw
  arc A14 (-135.136278, -155.760128) -> (-125.422656, -170.65176) centre (-122.682903, -158.250803) ccw
  line L19 (-135.136278, -155.760128) -> (-132.650594, -143.33171)
  arc A15 (-132.650594, -143.33171) -> (-133.08708, -141.339618) centre (-135.141269, -142.833575) ccw
  line L20 (-133.08708, -141.339618) -> (-152.034083, -115.287488)
  arc A16 (-152.425798, -113.108587) -> (-152.034083, -115.287488) centre (-149.979894, -113.793532) ccw
  line L21 (-152.425798, -113.108587) -> (-151.469892, -109.695095)
  arc A17 (-151.469892, -109.695095) -> (-21.748345, -130.644222) centre (-45.713045, 133.067717) ccw
  arc A18 (-21.748345, -130.644222) -> (-22.481496, -123.208852) centre (-22.860001, -127.000004) ccw
  arc A19 (-143.161124, -90.146177) -> (-22.481496, -123.208852) centre (-28.068159, 93.172915) ccw
  arc A20 (-144.804126, -85.891994) -> (-143.161124, -90.146177) centre (-141.135269, -86.919412) ccw
  line L22 (-144.804126, -85.891994) -> (-120.850229, -0.353884)
  line L23 (-120.850229, -0.353884) -> (-120.778095, -0.019779)
  arc A21 (-120.778095, -0.019779) -> (-139.828091, -0.007596) centre (-130.302156, 1.451354) ccw
  arc A22 (-139.828091, -0.007596) -> (-133.55128, 0.953733) centre (-136.689686, 0.473068) ccw
  arc A23 (-127.031955, 1.119355) -> (-133.55128, 0.953733) centre (-130.302156, 1.451354) ccw
  line L24 (-127.031955, 1.119355) -> (-158.54056, -111.396223)
  arc A24 (-158.54056, -111.396223) -> (-157.169557, -119.022379) centre (-149.979894, -113.793532) ccw
  line L25 (-157.169557, -119.022379) -> (-150.447427, -128.265308)
  arc A25 (-151.287777, -133.587526) -> (-150.447427, -128.265308) centre (-153.528712, -130.506242) ccw
  line L26 (-151.287777, -133.587526) -> (-161.231572, -140.819377)
  line L27 (-161.231572, -140.819377) -> (-161.30107, -140.667166)
  arc A26 (-160.020005, -127.000004) -> (10.16, -127.000004) centre (-74.930002, -111.760004) ccw
  arc A27 (-161.58264, -127.279879) -> (11.722635, -127.279879) centre (-74.930002, -111.760004) ccw
  line L28 (11.722635, -127.279879) -> (10.16, -127.000004)
  line L29 (-160.020005, -127.000004) -> (-161.58264, -127.279879)
  line L30 (-162.551383, -150.464332) -> (-153.542572, -158.111041)
  line L31 (-153.542572, -158.111041) -> (-152.752254, -157.480005)
  line L32 (-152.752254, -157.480005) -> (-159.912802, -148.512039)
  line L33 (9.700548, -148.512039) -> (2.54, -157.480005)
  line L34 (2.54, -157.480005) -> (3.330318, -158.111041)
  line L35 (3.330318, -158.111041) -> (12.339129, -150.464332)
  dimension "d45" = 1.5875
extrude "Extrude3" add sketch "Sketch12" along normal blind 25.4 and the other way blind 177.8 separate body contours L26 A26 A27 L29 | L3 L26 A26 A27 | L3 L8 A26 A27 | L8 L13 A26 A27 | L13 A26 A27 L28 picked at (-158.591439, -137.338878) picked at (-157.500967, -139.059668) picked at (-153.347357, -148.906552) picked at (7.572431, -139.266087) picked at (8.673914, -137.523853) makes body 3
sketch "Sketch13" plane through (0, 0, 0) normal (1, 0, 0) x (0, 0, -1)
  arc A0 (126.999998, -88.899999) -> (203.199997, -165.099998) centre (204.897168, -87.202828) ccw
  line L0 (126.999998, -88.899999) -> (114.300004, -88.899999)
  line L1 (114.300004, -88.899999) -> (114.300004, -177.800006)
  line L2 (114.300004, -177.800006) -> (203.200006, -177.800006)
  line L3 (203.200006, -177.800006) -> (203.199997, -165.099998)
  constraint horizontal L0
  constraint perpendicular L0 L1
  constraint perpendicular L1 L2
extrude "Extrude4" cut sketch "Sketch13" along normal blind -50.8 and the other way blind -292.1 bodies 3
fillet "Fillet1" radius 25.4 2 edges at (-10.941318, 31.496, -127.139941) (160.801322, 31.496, -127.139941) on bodies 3
sketch "Sketch14" plane through (0, 6.096, 0) normal (0, 1, 0) x (-1, 0, 0)
  line L0 (-161.30107, -140.667166) -> (-166.349343, -138.78378)
  line L1 (-166.349343, -138.78378) -> (-166.516315, -138.860017)
  line L2 (-166.516315, -138.860017) -> (-162.551383, -150.464332)
  line L3 (-159.912802, -148.512039) -> (-147.172342, -139.24625)
  arc A0 (-141.850124, -140.0866) -> (-147.172342, -139.24625) centre (-144.931408, -142.327534) ccw
  line L4 (-141.850124, -140.0866) -> (-139.204793, -143.72393)
  line L5 (-139.204793, -143.72393) -> (-141.362965, -154.51479)
  arc A1 (-141.362965, -154.51479) -> (-126.792533, -176.852239) centre (-122.682903, -158.250803) ccw
  arc A2 (-126.792533, -176.852239) -> (-23.419721, -176.852239) centre (-75.106127, 57.096199) ccw
  arc A3 (-23.419721, -176.852239) -> (-8.849289, -154.51479) centre (-27.52935, -158.250803) ccw
  line L6 (-8.849289, -154.51479) -> (-11.007461, -143.72393)
  line L7 (-11.007461, -143.72393) -> (-8.36213, -140.0866)
  arc A4 (-3.039912, -139.24625) -> (-8.36213, -140.0866) centre (-5.280846, -142.327534) ccw
  line L8 (-3.039912, -139.24625) -> (9.700548, -148.512039)
  line L9 (12.339129, -150.464332) -> (16.304061, -138.860017)
  line L10 (16.304061, -138.860017) -> (16.137089, -138.78378)
  line L11 (16.137089, -138.78378) -> (11.088816, -140.667166)
  line L12 (11.088816, -140.667166) -> (11.019318, -140.819377)
  line L13 (11.019318, -140.819377) -> (1.075524, -133.587526)
  arc A5 (0.235173, -128.265308) -> (1.075524, -133.587526) centre (3.316458, -130.506242) ccw
  line L14 (0.235173, -128.265308) -> (6.995717, -118.96956)
  arc A6 (6.995717, -118.96956) -> (8.366095, -111.341172) centre (-0.193946, -113.740713) ccw
  line L15 (8.366095, -111.341172) -> (-23.189622, 1.229628)
  arc A7 (-16.660973, 0.953733) -> (-23.189622, 1.229628) centre (-19.910098, 1.451354) ccw
  arc A8 (-16.660973, 0.953733) -> (-10.384163, -0.007596) centre (-13.522568, 0.473068) ccw
  arc A9 (-10.384163, -0.007596) -> (-29.434159, -0.019779) centre (-19.910098, 1.451354) ccw
  line L16 (-29.434159, -0.019779) -> (2.25178, -113.05513)
  arc A10 (1.860243, -115.234669) -> (2.25178, -113.05513) centre (-0.193946, -113.740713) ccw
  line L17 (1.860243, -115.234669) -> (-17.125174, -141.339618)
  arc A11 (-17.125174, -141.339618) -> (-17.56166, -143.33171) centre (-15.070985, -142.833575) ccw
  line L18 (-17.56166, -143.33171) -> (-15.075976, -155.760128)
  arc A12 (-24.789597, -170.65176) -> (-15.075976, -155.760128) centre (-27.52935, -158.250803) ccw
  arc A13 (-125.422656, -170.65176) -> (-24.789597, -170.65176) centre (-75.106127, 57.096199) ccw
  arc A14 (-135.136278, -155.760128) -> (-125.422656, -170.65176) centre (-122.682903, -158.250803) ccw
  line L19 (-135.136278, -155.760128) -> (-132.650594, -143.33171)
  arc A15 (-132.650594, -143.33171) -> (-133.08708, -141.339618) centre (-135.141269, -142.833575) ccw
  line L20 (-133.08708, -141.339618) -> (-152.034083, -115.287488)
  arc A16 (-152.425798, -113.108587) -> (-152.034083, -115.287488) centre (-149.979894, -113.793532) ccw
  line L21 (-152.425798, -113.108587) -> (-151.469892, -109.695095)
  arc A17 (-151.469892, -109.695095) -> (-21.748345, -130.644222) centre (-45.713045, 133.067717) ccw
  arc A18 (-21.748345, -130.644222) -> (-22.481496, -123.208852) centre (-22.860001, -127.000004) ccw
  arc A19 (-143.161124, -90.146177) -> (-22.481496, -123.208852) centre (-28.068159, 93.172915) ccw
  arc A20 (-144.804126, -85.891994) -> (-143.161124, -90.146177) centre (-141.135269, -86.919412) ccw
  line L22 (-144.804126, -85.891994) -> (-120.850229, -0.353884)
  line L23 (-120.850229, -0.353884) -> (-120.778095, -0.019779)
  arc A21 (-120.778095, -0.019779) -> (-139.828091, -0.007596) centre (-130.302156, 1.451354) ccw
  arc A22 (-139.828091, -0.007596) -> (-133.55128, 0.953733) centre (-136.689686, 0.473068) ccw
  arc A23 (-127.031955, 1.119355) -> (-133.55128, 0.953733) centre (-130.302156, 1.451354) ccw
  line L24 (-127.031955, 1.119355) -> (-158.54056, -111.396223)
  arc A24 (-158.54056, -111.396223) -> (-157.169557, -119.022379) centre (-149.979894, -113.793532) ccw
  line L25 (-157.169557, -119.022379) -> (-150.447427, -128.265308)
  arc A25 (-151.287777, -133.587526) -> (-150.447427, -128.265308) centre (-153.528712, -130.506242) ccw
  line L26 (-151.287777, -133.587526) -> (-161.231572, -140.819377)
  line L27 (-161.231572, -140.819377) -> (-161.30107, -140.667166)
  arc A26 (-126.792533, -176.852239) -> (-23.419721, -176.852239) centre (-75.106127, 57.096199) ccw
  line L28 (-75.106127, -182.493777) -> (-75.106127, -194.943676)
  arc A27 (-86.145404, -193.998332) -> (-64.07553, -194.058614) centre (-74.930002, -127.95861) ccw
  arc A28 (-85.354991, -199.487053) -> (-64.864679, -199.53855) centre (-74.930002, -127.95861) ccw
  line L29 (-78.281127, -182.493777) -> (-78.281127, -194.943676)
  line L30 (-71.931127, -182.493777) -> (-71.931127, -194.943676)
  line L31 (-64.864679, -199.53855) -> (-64.07553, -194.058614)
  line L32 (-85.347575, -199.53855) -> (-86.136723, -194.058614)
  line L33 (-86.136723, -194.058614) -> (-86.145404, -193.998332)
  line L34 (-71.931127, -182.493777) -> (-71.931127, -182.286349)
  line L35 (-71.931127, -182.286349) -> (-78.287735, -182.286349)
  line L36 (-78.287735, -182.286349) -> (-78.281127, -182.493777)
  line L37 (-162.551383, -150.464332) -> (-153.542572, -158.111041)
  line L38 (-153.542572, -158.111041) -> (-152.752254, -157.480005)
  line L39 (-152.752254, -157.480005) -> (-159.912802, -148.512039)
  line L40 (9.700548, -148.512039) -> (2.54, -157.480005)
  line L41 (2.54, -157.480005) -> (3.330318, -158.111041)
  line L42 (3.330318, -158.111041) -> (12.339129, -150.464332)
  dimension "d56" = 3.175
  dimension "d57" = -3.175
  constraint vertical L28
  constraint concentric A27 A28
  constraint parallel L32 L33
  constraint parallel L30 L34
  constraint perpendicular L34 L35
extrude "Extrude5" add sketch "Sketch14" against normal blind 6.096 separate body contours A2 A26 L28 A27 L29 L36 | A2 A26 L28 A27 L30 L34 | A27 A28 L31 L32 L33 picked at (-77.575893, -190.749698) picked at (-72.636539, -190.758984) picked at (-75.109686, -198.422112) makes body 4
combine "Combine1" operation add target body 2 tool bodies 4
chamfer "Chamfer3" distance 1.27 angle 45 2 edges at (64.07553, 3.048, -194.058614) (86.145404, 3.048, -193.998332) on bodies 2
chamfer "Chamfer4" distance 5.08 angle 45 2 edges at (85.354991, 3.048, -199.487053) (64.864679, 3.048, -199.53855) on bodies 2
fillet "Fillet2" radius 6.35 3 edges at (78.281127, 3.048, -182.493777) (78.281797, 3.048, -182.472729) (71.931127, 3.048, -182.472738) on bodies 2
sketch "Sketch15" plane through (159.413437, 0, -115.937045) normal (0.808736, 0, -0.588172) x (-0.588172, 0, -0.808736)
  line L0 (3.815007, 0) -> (15.243864, 0)
  line L1 (15.243864, 0) -> (15.243864, 6.096)
  line L2 (15.243864, 6.096) -> (3.815007, 6.096)
  line L3 (3.815007, 6.096) -> (3.815007, 0)
  line L4 (18.207999, 6.07946) -> (33.020001, 6.07946)
  line L5 (33.020001, 6.07946) -> (33.020001, -0.27054)
  line L6 (33.020001, -0.27054) -> (18.207999, -0.27054)
  line L7 (18.207999, -0.27054) -> (18.207999, 6.07946)
  dimension "d63" = 6.35
  constraint horizontal L4
  constraint vertical L5
  constraint horizontal L6
  constraint vertical L7
extrude "Extrude6" cut sketch "Sketch15" along normal blind 35.56 contours L4 L5 L6 L7 picked at (28.082667, 3.962794) bodies 3
sketch "Sketch16" plane through (0, 0, 0) normal (0, 0, 1) x (1, 0, 0)
  line L0 (79.305403, 6.149175) -> (70.929362, 6.149175)
  line L1 (75.117382, 6.149175) -> (75.117382, 0)
  line L2 (82.737382, 6.376587) -> (67.497382, 6.376587)
  line L3 (67.497382, 6.376587) -> (67.497382, -0.227413)
  line L4 (67.497382, -0.227413) -> (82.737382, -0.227413)
  line L5 (82.737382, -0.227413) -> (82.737382, 6.376587)
  line L6 (82.737382, 6.376587) -> (67.497382, -0.227413) construction
  line L7 (67.497382, 6.376587) -> (82.737382, -0.227413) construction
  point P0 (75.117382, 3.074587)
  dimension "d66" = 15.24
  dimension "d67" = 6.604
  constraint horizontal L0
  constraint perpendicular L0 L1
  constraint horizontal L2
  constraint perpendicular L2 L3
  constraint parallel L2 L4
  constraint parallel L3 L5
extrude "Extrude7" cut sketch "Sketch16" against normal blind 223.52 bodies 3
ref_plane "WorkPlane1" through (75.106127, 3.048, -98.051108) normal (1, 0, 0) x (0, 0, -1)